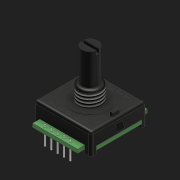
# Autodesk Inventor part: Bourns ACE 128
Saved by Autodesk Inventor 2017 SP1 (Build 210196100, 196)
## iProperties
Created: 2018-01-09
Part Number: Bourns ACE 128
Material: ABS Plastic
Document SubType Name: Modeling
Designer: Zach
Density: 1.06 g/cm^3
Appearance: Glossy - Black
Author: Zach
Autodesk Inventor part; units mm, degrees
ref_plane "YZ Plane" through (0, 0, 0) normal (1, 0, 0) x (0, 1, 0)
ref_plane "XZ Plane" through (0, 0, 0) normal (0, 1, 0) x (-1, 0, 0)
sketch "Sketch1" plane through (0, 0, 0) normal (0, 0, 1) x (1, 0, 0)
  line L0 (0, 0) -> (18.04, 0)
  line L1 (18.04, 0) -> (18.04, 27.94) construction
  line L2 (18.04, 27.94) -> (0, 27.94)
  line L3 (0, 27.94) -> (0, 0) construction
  circle A0 centre (9.02, 26.94) radius 0.32
  circle A1 centre (6.48, 26.94) radius 0.32
  circle A2 centre (3.94, 26.94) radius 0.32
  circle A3 centre (11.56, 26.94) radius 0.32
  circle A4 centre (14.1, 26.94) radius 0.32
  circle A5 centre (9.02, 1) radius 0.32
  circle A6 centre (6.48, 1) radius 0.32
  circle A7 centre (3.94, 1) radius 0.32
  circle A8 centre (11.56, 1) radius 0.32
  circle A9 centre (14.1, 1) radius 0.32
  line L4 (-2.665, 23.07) -> (20.705, 23.07) construction
  line L5 (20.705, 23.07) -> (20.705, 4.87) construction
  line L6 (20.705, 4.87) -> (-2.665, 4.87) construction
  line L7 (-2.665, 4.87) -> (-2.665, 23.07) construction
  line L8 (0, 27.94) -> (0, 23.07)
  line L9 (0, 23.07) -> (-2.665, 23.07)
  line L10 (-2.665, 23.07) -> (-2.665, 4.87)
  line L11 (-2.665, 4.87) -> (0, 4.87)
  line L12 (0, 0) -> (0, 4.87)
  line L13 (18.04, 0) -> (18.04, 4.87)
  line L14 (18.04, 4.87) -> (20.705, 4.87)
  line L15 (20.705, 4.87) -> (20.705, 23.07)
  line L16 (20.705, 23.07) -> (18.04, 23.07)
  line L17 (18.04, 23.07) -> (18.04, 27.94)
  point P0 (9.02, 27.94)
  point P1 (9.02, 23.07)
  point P2 (18.04, 13.97)
  point P3 (20.705, 13.97)
  dimension "d0" = 18.04
  dimension "d1" = 27.94
  dimension "d2" = 0.64
  dimension "d3" = 0.64
  dimension "d4" = 2.54
  dimension "d5" = 0.64
  dimension "d6" = 0.64
  dimension "d7" = 0.64
  dimension "d8" = 2.54
  dimension "d9" = 2.54
  dimension "d10" = 2.54
  dimension "d11" = 1
  dimension "d12" = 0.64
  dimension "d13" = 0.64
  dimension "d14" = 2.54
  dimension "d15" = 0.64
  dimension "d16" = 0.64
  dimension "d17" = 0.64
  dimension "d18" = 2.54
  dimension "d19" = 2.54
  dimension "d20" = 2.54
  dimension "d21" = 1
  dimension "d24" = 23.37
  dimension "d25" = 18.2
  constraints: 36 end point, 10 centre point, 9 horizontal alignment, 8 point on line, 4 collinear, 4 midpoint, 4 parallel, 4 perpendicular, 3 vertical alignment, 2 horizontal
  measures "d0" distance of L2.end L1.end
  measures "d1" distance of L1.end L0.end
  measures "d2" diameter of A0
  measures "d3" diameter of A1
  measures "d4" distance of A0.centre A1.centre
  measures "d5" diameter of A2
  measures "d6" diameter of A3
  measures "d7" diameter of A4
  measures "d8" distance of A3.centre A0.centre
  measures "d9" distance of A4.centre A3.centre
  measures "d10" distance of A2.centre A1.centre
  measures "d11" distance from line of L2 A2.centre
  measures "d12" diameter of A5
  measures "d13" diameter of A6
  measures "d14" distance of A5.centre A6.centre
  measures "d15" diameter of A7
  measures "d16" diameter of A8
  measures "d17" diameter of A9
  measures "d18" distance of A8.centre A5.centre
  measures "d19" distance of A9.centre A8.centre
  measures "d20" distance of A7.centre A6.centre
  measures "d21" distance from line of L0 A5.centre
  measures "d24" distance of L5.end L6.end
  measures "d25" distance of L4.end L5.end
extrude "Extrusion1" add sketch "Sketch1" along normal blind 1.5
sketch "Sketch2" plane through (0, 0, 1.5) normal (0, 0, 1) x (1, 0, 0)
  line L0 (-2.565, 25.07) -> (20.605, 25.07)
  line L1 (20.605, 25.07) -> (20.605, 2.87)
  line L2 (20.605, 2.87) -> (-2.565, 2.87)
  line L3 (-2.565, 2.87) -> (-2.565, 25.07)
  line L4 (-2.665, 23.07) -> (-2.665, 4.87) projected
  line L5 (20.705, 4.87) -> (20.705, 23.07) projected
  line L6 (18.04, 27.94) -> (0, 27.94) projected
  point P0 (0, 0)
  point P1 (9.02, 25.07)
  point P2 (9.02, 27.94)
  dimension "d27" = 22.2
  dimension "d30" = 0.1
  constraints: 8 end point, 2 midpoint, 2 parallel, 1 horizontal, 1 perpendicular, 1 vertical alignment
  measures "d27" distance of L0.end L1.end
  measures "d30" distance between parallel lines of L5 L1
extrude "Extrusion2" add sketch "Sketch2" along normal blind 5.51
sketch "Sketch3" plane through (0, 0, 1.5) normal (0, 0, -1) x (-1, 0, 0)
  line L0 (0, 23.07) -> (2.565, 23.07) projected
  line L1 (2.565, 23.07) -> (2.565, 25.07) projected
  line L2 (2.565, 25.07) -> (0, 25.07) projected
  line L3 (0, 25.07) -> (0, 23.07) projected
  line L4 (0, 4.87) -> (0, 2.87) projected
  line L5 (0, 2.87) -> (2.565, 2.87) projected
  line L6 (2.565, 2.87) -> (2.565, 4.87) projected
  line L7 (2.565, 4.87) -> (0, 4.87) projected
  line L8 (-20.605, 23.07) -> (-18.04, 23.07) projected
  line L9 (-18.04, 23.07) -> (-18.04, 25.07) projected
  line L10 (-18.04, 25.07) -> (-20.605, 25.07) projected
  line L11 (-20.605, 25.07) -> (-20.605, 23.07) projected
  line L12 (-18.04, 2.87) -> (-18.04, 4.87) projected
  line L13 (-18.04, 4.87) -> (-20.605, 4.87) projected
  line L14 (-20.605, 4.87) -> (-20.605, 2.87) projected
  line L15 (-20.605, 2.87) -> (-18.04, 2.87) projected
  point P0 (0, 0)
extrude "Extrusion3" add sketch "Sketch3" along normal blind 3
sketch "Sketch4" plane through (0, 0, 7.01) normal (0, 0, 1) x (1, 0, 0)
  circle A0 centre (9.02, 13.97) radius 4.5
  line L0 (20.605, 25.07) -> (-2.565, 25.07) construction
  line L1 (-2.565, 25.07) -> (-2.565, 2.87) construction
  line L2 (-2.565, 2.87) -> (20.605, 2.87) construction
  line L3 (20.605, 2.87) -> (20.605, 25.07) construction
  point P0 (0, 0)
  point P1 (9.02, 25.07)
  point P2 (20.605, 13.97)
  dimension "d33" = 9
  constraints: 2 midpoint, 1 centre point, 1 horizontal alignment, 1 vertical alignment
  measures "d33" diameter of A0
extrude "Extrusion4" add sketch "Sketch4" along normal blind 6.35
sketch "Sketch5" plane through (9.02, 13.97, 13.36) normal (0, 0, 1) x (1, 0, 0)
  circle A0 centre (0, 0) radius 3.16
  circle A1 centre (0, 0) radius 4.5 construction
  point P0 (-9.02, -13.97)
  dimension "d36" = 6.32
  constraints: 1 centre point, 1 coincident
  measures "d36" diameter of A0
extrude "Extrusion5" add sketch "Sketch5" along normal blind 12.7
sketch "Sketch6" plane through (9.02, 13.97, 26.06) normal (0, 0, 1) x (1, 0, 0)
  line L0 (-3.16, 0.595) -> (3.16, 0.595)
  line L1 (3.16, 0.595) -> (3.16, -0.595)
  line L2 (3.16, -0.595) -> (-3.16, -0.595)
  line L3 (-3.16, -0.595) -> (-3.16, 0.595)
  circle A0 centre (0, 0) radius 3.16 construction
  point P0 (-9.02, -13.97)
  point P1 (3.16, 0)
  point P2 (0, 0.595)
  dimension "d39" = 1.19
  constraints: 8 end point, 2 horizontal alignment, 2 midpoint, 2 parallel, 1 horizontal, 1 perpendicular, 1 vertical alignment, 1 other
  measures "d39" distance of L0.end L1.end
extrude "Extrusion6" cut sketch "Sketch6" against normal blind 1.6
thread "Thread1" size "M9x1.25" class "6g" standard "ANSI Metric M Profile" full length
fillet "Fillet1" radius 1 1 edges at (4.52, 13.97, 13.36)
fillet "Fillet2" radius 1 4 edges at (20.605, 2.87, 2.755) (-2.565, 2.87, 2.755) (-2.565, 25.07, 2.755) (20.605, 25.07, 2.755)
fillet "Fillet3" radius 1 8 edges at (-2.2721, 24.7771, 7.01) (-2.565, 13.97, 7.01) (-2.2721, 3.1629, 7.01) (9.02, 2.87, 7.01) (20.3121, 3.1629, 7.01) (20.605, 13.97, 7.01) (20.3121, 24.7771, 7.01) (9.02, 25.07, 7.01)
ref_plane "Work Plane1" through (0, 13.97, 1.5) normal (0, 1, 0) x (1, 0, 0)
sketch "Sketch8" plane through (0, 13.97, 1.5) normal (0, 1, 0) x (1, 0, 0)
  line L0 (19.605, -1.51) -> (21.605, -1.51)
  line L1 (19.605, 3) -> (19.605, -4.51) construction
  line L2 (19.605, -1.51) -> (19.605, -5.51)
  line L3 (0, 1.5) -> (18.04, 1.5) construction
  line L4 (9.02, 1.5) -> (9.02, -5.51) construction
  line L5 (19.605, -5.51) -> (-1.565, -5.51) construction
  line L6 (21.605, -1.51) -> (19.605, -5.51)
  line L7 (-1.565, -1.51) -> (-3.565, -1.51)
  line L8 (-1.565, -1.51) -> (-1.565, -5.51)
  line L9 (-3.565, -1.51) -> (-1.565, -5.51)
  dimension "d47" = 2
  dimension "d48" = 4
  constraints: 14 end point, 3 symmetric about line, 2 vertical, 1 horizontal, 1 midpoint, 1 point on line
  measures "d47" distance of L0.start L0.end
  measures "d48" distance of L2.end L0.start
extrude "Extrusion7" add sketch "Sketch8" along normal mid plane 2.79
sketch "Sketch9" plane through (0, 13.97, 1.5) normal (0, 1, 0) x (1, 0, 0)
  line L0 (-1.565, -5.51) -> (19.605, -5.51) projected
  line L1 (19.605, -5.51) -> (18.415, -5.51)
  line L2 (18.415, -5.51) -> (18.415, -7.03)
  line L3 (18.415, -7.03) -> (19.605, -7.03)
  line L4 (19.605, -7.03) -> (19.605, -5.51)
  point P0 (0, 1.5)
  dimension "d51" = 1.52
  dimension "d52" = 1.19
  constraints: 8 end point, 2 parallel, 1 horizontal, 1 perpendicular
  measures "d51" distance of L2.end L1.end
  measures "d52" distance of L2.end L3.end
extrude "Extrusion8" add sketch "Sketch9" along normal mid plane 2.79
sketch "Sketch10" plane through (0, 0, 7.01) normal (0, 0, 1) x (1, 0, 0)
  circle A0 centre (9.02, 13.97) radius 4.5 projected
  circle A1 centre (9.02, 13.97) radius 7.35
  point P0 (0, 0)
  dimension "d55" = 14.7
  constraints: 1 centre point, 1 coincident
  measures "d55" diameter of A1
extrude "Extrusion9" add sketch "Sketch10" along normal blind 0.25 contours A0 | A1
sketch "Sketch11" plane through (0, 0, 1.5) normal (0, 0, 1) x (1, 0, 0)
  circle A0 centre (9.02, 1) radius 0.32 projected
  circle A1 centre (6.48, 1) radius 0.32 projected
  circle A2 centre (3.94, 1) radius 0.32 projected
  circle A3 centre (11.56, 1) radius 0.32 projected
  circle A4 centre (14.1, 1) radius 0.32 projected
  line L0 (18.04, 2.87) -> (0, 2.87) projected
  line L1 (0, 2.87) -> (0, 0) construction
  line L2 (0, 0) -> (18.04, 0) construction
  line L3 (18.04, 0) -> (18.04, 2.87) construction
  circle A5 centre (9.02, 26.94) radius 0.32 projected
  circle A6 centre (6.48, 26.94) radius 0.32 projected
  circle A7 centre (3.94, 26.94) radius 0.32 projected
  circle A8 centre (11.56, 26.94) radius 0.32 projected
  circle A9 centre (14.1, 26.94) radius 0.32 projected
  line L4 (0, 25.07) -> (18.04, 25.07) construction
  line L5 (18.04, 25.07) -> (18.04, 27.94) construction
  line L6 (18.04, 27.94) -> (0, 27.94) construction
  line L7 (0, 27.94) -> (0, 25.07) construction
extrude "Extrusion10" add sketch "Sketch11" along normal blind 1 and the other way blind 6.5
sketch "Sketch12" plane through (0, 0, 7.01) normal (0, 0, 1) x (1, 0, 0)
  line L0 (16.6233, 23.2524) -> (16.6233, 21.4375) construction
  line L1 (16.6233, 21.4375) -> (0.9162, 21.4375) construction
  line L2 (0.9162, 21.4375) -> (0.9162, 23.2524) construction
  line L3 (0.9162, 23.2524) -> (16.6233, 23.2524) construction
  line L4 (16.6326, 7.0655) -> (16.6326, 4.3638) construction
  line L5 (16.6326, 4.3638) -> (0.3771, 4.3638) construction
  line L6 (0.3771, 4.3638) -> (0.3771, 7.0655) construction
  line L7 (0.3771, 7.0655) -> (16.6326, 7.0655) construction
  line L8 (14.592, 6.0867) -> (14.592, 7.0623)
  line L9 (14.592, 7.0623) -> (14.7963, 7.0623)
  line L10 (14.7963, 7.0623) -> (14.7963, 6.6993)
  line L11 (14.7963, 6.6993) -> (16.1366, 6.6993)
  line L12 (16.1366, 6.6993) -> (16.1366, 7.0623)
  line L13 (16.1366, 7.0623) -> (16.3198, 7.0623)
  spline S0 degree 2 poles (16.3198, 7.0623) (16.3198, 6.8565) (16.4365, 6.662) (16.5985, 6.6491) knots 0 0 0 1 2 2 2
  line L14 (16.5985, 6.6491) -> (16.5985, 6.4416)
  line L15 (16.5985, 6.4416) -> (14.7963, 6.4416)
  line L16 (14.7963, 6.4416) -> (14.7963, 6.0867)
  line L17 (14.7963, 6.0867) -> (14.592, 6.0867)
  spline S1 degree 2 poles (15.592, 4.474) (15.054, 4.474) (14.5499, 4.7868) (14.5499, 5.1126) knots 0 0 0 1 2 2 2
  spline S2 degree 2 poles (14.5499, 5.1126) (14.5499, 5.4432) (15.0637, 5.7528) (15.5904, 5.7528) knots 0 0 0 1 2 2 2
  spline S3 degree 2 poles (15.5904, 5.7528) (16.1318, 5.7528) (16.6326, 5.44) (16.6326, 5.1126) knots 0 0 0 1 2 2 2
  spline S4 degree 2 poles (16.6326, 5.1126) (16.6326, 4.7836) (16.1139, 4.474) (15.592, 4.474) knots 0 0 0 1 2 2 2
  spline S5 degree 2 poles (14.9826, 4.8176) (15.0815, 4.7787) (15.3862, 4.7463) (15.592, 4.7463) knots 0 0 0 1 2 2 2
  spline S6 degree 2 poles (15.592, 4.7463) (15.7979, 4.7463) (16.101, 4.7787) (16.2031, 4.8192) knots 0 0 0 1 2 2 2
  spline S7 degree 2 poles (16.2031, 4.8192) (16.3052, 4.8598) (16.4105, 5.0008) (16.4105, 5.1126) knots 0 0 0 1 2 2 2
  spline S8 degree 2 poles (16.4105, 5.1126) (16.4105, 5.2244) (16.3052, 5.3687) (16.1998, 5.4108) knots 0 0 0 1 2 2 2
  spline S9 degree 2 poles (16.1998, 5.4108) (16.0977, 5.4513) (15.7865, 5.4805) (15.5904, 5.4805) knots 0 0 0 1 2 2 2
  spline S10 degree 2 poles (15.5904, 5.4805) (15.3797, 5.4805) (15.0977, 5.4546) (14.9875, 5.4124) knots 0 0 0 1 2 2 2
  spline S11 degree 2 poles (14.9875, 5.4124) (14.8838, 5.3735) (14.7719, 5.2293) (14.7719, 5.1126) knots 0 0 0 1 2 2 2
  spline S12 degree 2 poles (14.7719, 5.1126) (14.7719, 5.0024) (14.8773, 4.8581) (14.9826, 4.8176) knots 0 0 0 1 2 2 2
  spline S13 degree 2 poles (12.6492, 5.7739) (12.8031, 5.7739) (13.0592, 5.6734) (13.1516, 5.5858) knots 0 0 0 1 2 2 2
  spline S14 degree 2 poles (13.1516, 5.5858) (13.2407, 5.5032) (13.3396, 5.2617) (13.3396, 5.1385) knots 0 0 0 1 2 2 2
  spline S15 degree 2 poles (13.3396, 5.1385) (13.3396, 5.0008) (13.2472, 4.7771) (13.1597, 4.6944) knots 0 0 0 1 2 2 2
  spline S16 degree 2 poles (13.1597, 4.6944) (13.0495, 4.5907) (12.6929, 4.4773) (12.419, 4.4773) knots 0 0 0 1 2 2 2
  spline S17 degree 2 poles (12.419, 4.4773) (12.1711, 4.4773) (11.727, 4.5891) (11.5795, 4.6977) knots 0 0 0 1 2 2 2
  spline S18 degree 2 poles (11.5795, 4.6977) (11.4239, 4.8127) (11.2602, 5.1369) (11.2602, 5.3735) knots 0 0 0 1 2 2 2
  spline S19 degree 2 poles (11.2602, 5.3735) (11.2602, 5.427) (11.2715, 5.5486) (11.2877, 5.6004) knots 0 0 0 1 2 2 2
  line L18 (11.2877, 5.6004) -> (11.5454, 5.6004)
  line L19 (11.5454, 5.6004) -> (11.5454, 5.5875)
  spline S20 degree 2 poles (11.5454, 5.5875) (11.526, 5.5534) (11.492, 5.4108) (11.492, 5.3379) knots 0 0 0 1 2 2 2
  spline S21 degree 2 poles (11.492, 5.3379) (11.492, 5.0753) (11.8388, 4.7755) (12.1597, 4.7544) knots 0 0 0 1 2 2 2
  spline S22 degree 2 poles (12.1597, 4.7544) (12.0868, 4.8614) (12.0203, 5.0559) (12.0203, 5.1709) knots 0 0 0 1 2 2 2
  spline S23 degree 2 poles (12.0203, 5.1709) (12.0203, 5.2811) (12.0689, 5.4643) (12.1386, 5.5567) knots 0 0 0 1 2 2 2
  spline S24 degree 2 poles (12.1386, 5.5567) (12.2213, 5.6636) (12.4725, 5.7739) (12.6492, 5.7739) knots 0 0 0 1 2 2 2
  spline S25 degree 2 poles (12.479, 4.7479) (12.6816, 4.7479) (12.9377, 4.8225) (13.0074, 4.8889) knots 0 0 0 1 2 2 2
  spline S26 degree 2 poles (13.0074, 4.8889) (13.0722, 4.9473) (13.1208, 5.0688) (13.1208, 5.1401) knots 0 0 0 1 2 2 2
  spline S27 degree 2 poles (13.1208, 5.1401) (13.1208, 5.3055) (12.8842, 5.5016) (12.6605, 5.5016) knots 0 0 0 1 2 2 2
  spline S28 degree 2 poles (12.6605, 5.5016) (12.5341, 5.5016) (12.3704, 5.4367) (12.3121, 5.3654) knots 0 0 0 1 2 2 2
  spline S29 degree 2 poles (12.3121, 5.3654) (12.2699, 5.3136) (12.2424, 5.1855) (12.2424, 5.111) knots 0 0 0 1 2 2 2
  spline S30 degree 2 poles (12.2424, 5.111) (12.2424, 5.0251) (12.3023, 4.8273) (12.3526, 4.7528) knots 0 0 0 1 2 2 2
  spline S31 degree 2 poles (12.3526, 4.7528) (12.372, 4.7512) (12.4385, 4.7479) (12.479, 4.7479) knots 0 0 0 1 2 2 2
  spline S32 degree 2 poles (7.9608, 5.1142) (7.9608, 5.2633) (8.0499, 5.508) (8.1326, 5.5939) knots 0 0 0 1 2 2 2
  spline S33 degree 2 poles (8.1326, 5.5939) (8.2136, 5.6782) (8.434, 5.7657) (8.5588, 5.7657) knots 0 0 0 1 2 2 2
  spline S34 degree 2 poles (8.5588, 5.7657) (8.7209, 5.7657) (8.9932, 5.5923) (9.0742, 5.427) knots 0 0 0 1 2 2 2
  line L20 (9.0742, 5.427) -> (9.0823, 5.427)
  spline S35 degree 2 poles (9.0823, 5.427) (9.1682, 5.5745) (9.3724, 5.7171) (9.5248, 5.7171) knots 0 0 0 1 2 2 2
  spline S36 degree 2 poles (9.5248, 5.7171) (9.7501, 5.7171) (10.0515, 5.3768) (10.0515, 5.1142) knots 0 0 0 1 2 2 2
  spline S37 degree 2 poles (10.0515, 5.1142) (10.0515, 4.8419) (9.7663, 4.5129) (9.5426, 4.5129) knots 0 0 0 1 2 2 2
  spline S38 degree 2 poles (9.5426, 4.5129) (9.4081, 4.5129) (9.1455, 4.6701) (9.071, 4.8176) knots 0 0 0 1 2 2 2
  line L21 (9.071, 4.8176) -> (9.0629, 4.8176)
  spline S39 degree 2 poles (9.0629, 4.8176) (8.9818, 4.6426) (8.7484, 4.4627) (8.5637, 4.4627) knots 0 0 0 1 2 2 2
  spline S40 degree 2 poles (8.5637, 4.4627) (8.3076, 4.4627) (7.9608, 4.8354) (7.9608, 5.1142) knots 0 0 0 1 2 2 2
  spline S41 degree 2 poles (8.5378, 4.7382) (8.6609, 4.7382) (8.8068, 4.8354) (8.8814, 4.9732) knots 0 0 0 1 2 2 2
  spline S42 degree 2 poles (8.8814, 4.9732) (8.9073, 5.0186) (8.9673, 5.1709) (9.0061, 5.2666) knots 0 0 0 1 2 2 2
  spline S43 degree 2 poles (9.0061, 5.2666) (8.9332, 5.3768) (8.716, 5.4951) (8.5783, 5.4951) knots 0 0 0 1 2 2 2
  spline S44 degree 2 poles (8.5783, 5.4951) (8.3967, 5.4951) (8.1601, 5.2763) (8.1601, 5.111) knots 0 0 0 1 2 2 2
  spline S45 degree 2 poles (8.1601, 5.111) (8.1601, 4.9424) (8.3627, 4.7382) (8.5378, 4.7382) knots 0 0 0 1 2 2 2
  spline S46 degree 2 poles (9.5394, 4.7755) (9.6739, 4.7755) (9.8538, 4.9554) (9.8538, 5.1158) knots 0 0 0 1 2 2 2
  spline S47 degree 2 poles (9.8538, 5.1158) (9.8538, 5.2617) (9.6933, 5.4481) (9.5556, 5.4481) knots 0 0 0 1 2 2 2
  spline S48 degree 2 poles (9.5556, 5.4481) (9.4567, 5.4481) (9.319, 5.3525) (9.2638, 5.2568) knots 0 0 0 1 2 2 2
  spline S49 degree 2 poles (9.2638, 5.2568) (9.2412, 5.2163) (9.1617, 5.0445) (9.139, 4.9748) knots 0 0 0 1 2 2 2
  spline S50 degree 2 poles (9.139, 4.9748) (9.2282, 4.8581) (9.4178, 4.7755) (9.5394, 4.7755) knots 0 0 0 1 2 2 2
  line L22 (6.4134, 4.4627) -> (4.7132, 5.3281)
  line L23 (4.7132, 5.3281) -> (4.7132, 5.6134)
  line L24 (4.7132, 5.6134) -> (6.4782, 4.6993)
  line L25 (6.4782, 4.6993) -> (6.4782, 5.7317)
  line L26 (6.4782, 5.7317) -> (6.7132, 5.7317)
  line L27 (6.7132, 5.7317) -> (6.7132, 4.4627)
  line L28 (6.7132, 4.4627) -> (6.4134, 4.4627)
  spline S51 degree 2 poles (2.0686, 4.4546) (1.9146, 4.4546) (1.6536, 4.5567) (1.5661, 4.6426) knots 0 0 0 1 2 2 2
  spline S52 degree 2 poles (1.5661, 4.6426) (1.4737, 4.7317) (1.3781, 4.9554) (1.3781, 5.0899) knots 0 0 0 1 2 2 2
  spline S53 degree 2 poles (1.3781, 5.0899) (1.3781, 5.2244) (1.4689, 5.4465) (1.5596, 5.5307) knots 0 0 0 1 2 2 2
  spline S54 degree 2 poles (1.5596, 5.5307) (1.6682, 5.6345) (2.0329, 5.7512) (2.2987, 5.7512) knots 0 0 0 1 2 2 2
  spline S55 degree 2 poles (2.2987, 5.7512) (2.5596, 5.7512) (2.9794, 5.6442) (3.135, 5.5324) knots 0 0 0 1 2 2 2
  spline S56 degree 2 poles (3.135, 5.5324) (3.2874, 5.4238) (3.4575, 5.0802) (3.4575, 4.8549) knots 0 0 0 1 2 2 2
  spline S57 degree 2 poles (3.4575, 4.8549) (3.4575, 4.7884) (3.4446, 4.6717) (3.43, 4.628) knots 0 0 0 1 2 2 2
  line L29 (3.43, 4.628) -> (3.1723, 4.628)
  line L30 (3.1723, 4.628) -> (3.1723, 4.6393)
  spline S58 degree 2 poles (3.1723, 4.6393) (3.1917, 4.6766) (3.2258, 4.8127) (3.2258, 4.8905) knots 0 0 0 1 2 2 2
  spline S59 degree 2 poles (3.2258, 4.8905) (3.2258, 5.1401) (2.8886, 5.4465) (2.558, 5.4756) knots 0 0 0 1 2 2 2
  spline S60 degree 2 poles (2.558, 5.4756) (2.6245, 5.38) (2.6974, 5.179) (2.6974, 5.0591) knots 0 0 0 1 2 2 2
  spline S61 degree 2 poles (2.6974, 5.0591) (2.6974, 4.9424) (2.6504, 4.7674) (2.5791, 4.6717) knots 0 0 0 1 2 2 2
  spline S62 degree 2 poles (2.5791, 4.6717) (2.4964, 4.5615) (2.2404, 4.4546) (2.0686, 4.4546) knots 0 0 0 1 2 2 2
  spline S63 degree 2 poles (2.0572, 4.7269) (2.1804, 4.7269) (2.3473, 4.7917) (2.4057, 4.863) knots 0 0 0 1 2 2 2
  spline S64 degree 2 poles (2.4057, 4.863) (2.4478, 4.9165) (2.4754, 5.0494) (2.4754, 5.1191) knots 0 0 0 1 2 2 2
  spline S65 degree 2 poles (2.4754, 5.1191) (2.4754, 5.2131) (2.4186, 5.3897) (2.3651, 5.4756) knots 0 0 0 1 2 2 2
  spline S66 degree 2 poles (2.3651, 5.4756) (2.336, 5.4773) (2.2809, 5.4805) (2.2387, 5.4805) knots 0 0 0 1 2 2 2
  spline S67 degree 2 poles (2.2387, 5.4805) (2.0313, 5.4805) (1.7768, 5.3995) (1.7104, 5.3379) knots 0 0 0 1 2 2 2
  spline S68 degree 2 poles (1.7104, 5.3379) (1.6472, 5.2811) (1.5969, 5.158) (1.5969, 5.0883) knots 0 0 0 1 2 2 2
  spline S69 degree 2 poles (1.5969, 5.0883) (1.5969, 4.9262) (1.8271, 4.7269) (2.0572, 4.7269) knots 0 0 0 1 2 2 2
  line L31 (14.6168, 21.9736) -> (14.6168, 22.9493)
  line L32 (14.6168, 22.9493) -> (14.821, 22.9493)
  line L33 (14.821, 22.9493) -> (14.821, 22.5863)
  line L34 (14.821, 22.5863) -> (16.1614, 22.5863)
  line L35 (16.1614, 22.5863) -> (16.1614, 22.9493)
  line L36 (16.1614, 22.9493) -> (16.3445, 22.9493)
  spline S70 degree 2 poles (16.3445, 22.9493) (16.3445, 22.7435) (16.4612, 22.549) (16.6233, 22.536) knots 0 0 0 1 2 2 2
  line L37 (16.6233, 22.536) -> (16.6233, 22.3286)
  line L38 (16.6233, 22.3286) -> (14.821, 22.3286)
  line L39 (14.821, 22.3286) -> (14.821, 21.9736)
  line L40 (14.821, 21.9736) -> (14.6168, 21.9736)
  line L41 (11.3238, 21.8731) -> (11.3238, 23.1065)
  line L42 (11.3238, 23.1065) -> (11.6075, 23.1065)
  spline S71 degree 2 poles (11.6075, 23.1065) (11.7323, 22.9736) (11.964, 22.737) (12.0888, 22.6236) knots 0 0 0 1 2 2 2
  spline S72 degree 2 poles (12.0888, 22.6236) (12.34, 22.395) (12.6415, 22.2281) (12.802, 22.2281) knots 0 0 0 1 2 2 2
  spline S73 degree 2 poles (12.802, 22.2281) (12.8862, 22.2281) (13.0127, 22.28) (13.0532, 22.327) knots 0 0 0 1 2 2 2
  spline S74 degree 2 poles (13.0532, 22.327) (13.0937, 22.374) (13.1342, 22.4971) (13.1342, 22.5717) knots 0 0 0 1 2 2 2
  spline S75 degree 2 poles (13.1342, 22.5717) (13.1342, 22.643) (13.0986, 22.7889) (13.071, 22.8553) knots 0 0 0 1 2 2 2
  spline S76 degree 2 poles (13.071, 22.8553) (13.0483, 22.912) (12.9835, 23.0174) (12.9608, 23.0498) knots 0 0 0 1 2 2 2
  line L43 (12.9608, 23.0498) -> (12.9608, 23.0644)
  line L44 (12.9608, 23.0644) -> (13.246, 23.0644)
  spline S77 degree 2 poles (13.246, 23.0644) (13.2866, 22.9817) (13.366, 22.6851) (13.366, 22.5522) knots 0 0 0 1 2 2 2
  spline S78 degree 2 poles (13.366, 22.5522) (13.366, 22.2718) (13.0694, 21.9558) (12.8165, 21.9558) knots 0 0 0 1 2 2 2
  spline S79 degree 2 poles (12.8165, 21.9558) (12.6982, 21.9558) (12.5005, 22.0109) (12.4162, 22.0595) knots 0 0 0 1 2 2 2
  spline S80 degree 2 poles (12.4162, 22.0595) (12.3287, 22.1082) (12.1569, 22.2492) (12.0742, 22.327) knots 0 0 0 1 2 2 2
  spline S81 degree 2 poles (12.0742, 22.327) (11.9365, 22.4534) (11.6415, 22.7629) (11.5556, 22.8553) knots 0 0 0 1 2 2 2
  line L45 (11.5556, 22.8553) -> (11.5556, 21.8731)
  line L46 (11.5556, 21.8731) -> (11.3238, 21.8731)
  spline S82 degree 2 poles (9.8413, 22.5668) (9.8413, 22.6398) (9.8056, 22.784) (9.7781, 22.8537) knots 0 0 0 1 2 2 2
  spline S83 degree 2 poles (9.7781, 22.8537) (9.7505, 22.9185) (9.6922, 23.0142) (9.6662, 23.0514) knots 0 0 0 1 2 2 2
  line L47 (9.6662, 23.0514) -> (9.6662, 23.0676)
  line L48 (9.6662, 23.0676) -> (9.9498, 23.0676)
  spline S84 degree 2 poles (9.9498, 23.0676) (9.9969, 22.9801) (10.073, 22.6803) (10.073, 22.5458) knots 0 0 0 1 2 2 2
  spline S85 degree 2 poles (10.073, 22.5458) (10.073, 22.4096) (10.0179, 22.207) (9.9596, 22.1244) knots 0 0 0 1 2 2 2
  spline S86 degree 2 poles (9.9596, 22.1244) (9.8964, 22.0368) (9.7132, 21.9461) (9.59, 21.9461) knots 0 0 0 1 2 2 2
  spline S87 degree 2 poles (9.59, 21.9461) (9.4247, 21.9461) (9.1751, 22.1633) (9.1427, 22.3156) knots 0 0 0 1 2 2 2
  line L49 (9.1427, 22.3156) -> (9.1233, 22.3156)
  spline S88 degree 2 poles (9.1233, 22.3156) (9.1103, 22.2524) (9.052, 22.1082) (8.9936, 22.0466) knots 0 0 0 1 2 2 2
  spline S89 degree 2 poles (8.9936, 22.0466) (8.9369, 21.985) (8.7554, 21.9072) (8.6241, 21.9072) knots 0 0 0 1 2 2 2
  spline S90 degree 2 poles (8.6241, 21.9072) (8.4896, 21.9072) (8.261, 21.9996) (8.1735, 22.0838) knots 0 0 0 1 2 2 2
  spline S91 degree 2 poles (8.1735, 22.0838) (8.0828, 22.1714) (7.9887, 22.4193) (7.9887, 22.5765) knots 0 0 0 1 2 2 2
  spline S92 degree 2 poles (7.9887, 22.5765) (7.9887, 22.7273) (8.0617, 23.0223) (8.1119, 23.1227) knots 0 0 0 1 2 2 2
  line L50 (8.1119, 23.1227) -> (8.3956, 23.1227)
  line L51 (8.3956, 23.1227) -> (8.3956, 23.1033)
  spline S93 degree 2 poles (8.3956, 23.1033) (8.334, 23.019) (8.2205, 22.7338) (8.2205, 22.5928) knots 0 0 0 1 2 2 2
  spline S94 degree 2 poles (8.2205, 22.5928) (8.2205, 22.5101) (8.2724, 22.3448) (8.3323, 22.2897) knots 0 0 0 1 2 2 2
  spline S95 degree 2 poles (8.3323, 22.2897) (8.3923, 22.2362) (8.5349, 22.1795) (8.6435, 22.1795) knots 0 0 0 1 2 2 2
  spline S96 degree 2 poles (8.6435, 22.1795) (8.7521, 22.1795) (8.8931, 22.2427) (8.9336, 22.2994) knots 0 0 0 1 2 2 2
  spline S97 degree 2 poles (8.9336, 22.2994) (8.9742, 22.3561) (9.005, 22.5101) (9.005, 22.6009) knots 0 0 0 1 2 2 2
  line L52 (9.005, 22.6009) -> (9.005, 22.7143)
  line L53 (9.005, 22.7143) -> (9.227, 22.7143)
  line L54 (9.227, 22.7143) -> (9.227, 22.6252)
  spline S98 degree 2 poles (9.227, 22.6252) (9.227, 22.4453) (9.3988, 22.2184) (9.5625, 22.2184) knots 0 0 0 1 2 2 2
  spline S99 degree 2 poles (9.5625, 22.2184) (9.6387, 22.2184) (9.7473, 22.2767) (9.7797, 22.3237) knots 0 0 0 1 2 2 2
  spline S100 degree 2 poles (9.7797, 22.3237) (9.8137, 22.374) (9.8413, 22.4971) (9.8413, 22.5668) knots 0 0 0 1 2 2 2
  line L55 (5.4251, 21.8197) -> (5.4251, 22.0579)
  line L56 (5.4251, 22.0579) -> (4.7379, 22.0579)
  line L57 (4.7379, 22.0579) -> (4.7379, 22.3156)
  line L58 (4.7379, 22.3156) -> (5.4251, 22.3156)
  line L59 (5.4251, 22.3156) -> (5.4251, 23.1989)
  line L60 (5.4251, 23.1989) -> (5.7071, 23.1989)
  line L61 (5.7071, 23.1989) -> (6.7379, 22.3043)
  line L62 (6.7379, 22.3043) -> (6.7379, 22.0579)
  line L63 (6.7379, 22.0579) -> (5.6407, 22.0579)
  line L64 (5.6407, 22.0579) -> (5.6407, 21.8197)
  line L65 (5.6407, 21.8197) -> (5.4251, 21.8197)
  line L66 (5.6407, 22.3156) -> (6.4219, 22.3156)
  line L67 (6.4219, 22.3156) -> (5.6407, 22.9882)
  line L68 (5.6407, 22.9882) -> (5.6407, 22.3156)
  spline S101 degree 2 poles (2.0803, 21.8942) (1.9361, 21.8942) (1.6897, 21.9866) (1.599, 22.0709) knots 0 0 0 1 2 2 2
  spline S102 degree 2 poles (1.599, 22.0709) (1.5082, 22.1552) (1.4029, 22.4064) (1.4029, 22.562) knots 0 0 0 1 2 2 2
  spline S103 degree 2 poles (1.4029, 22.562) (1.4029, 22.7046) (1.4661, 22.9834) (1.5163, 23.0855) knots 0 0 0 1 2 2 2
  line L69 (1.5163, 23.0855) -> (1.7999, 23.0855)
  line L70 (1.7999, 23.0855) -> (1.7999, 23.066)
  spline S104 degree 2 poles (1.7999, 23.066) (1.7772, 23.0352) (1.7189, 22.9201) (1.693, 22.8505) knots 0 0 0 1 2 2 2
  spline S105 degree 2 poles (1.693, 22.8505) (1.6654, 22.771) (1.6346, 22.6398) (1.6346, 22.5571) knots 0 0 0 1 2 2 2
  spline S106 degree 2 poles (1.6346, 22.5571) (1.6346, 22.4761) (1.693, 22.3237) (1.7562, 22.2686) knots 0 0 0 1 2 2 2
  spline S107 degree 2 poles (1.7562, 22.2686) (1.8161, 22.2184) (1.975, 22.1665) (2.0819, 22.1665) knots 0 0 0 1 2 2 2
  spline S108 degree 2 poles (2.0819, 22.1665) (2.1889, 22.1665) (2.3251, 22.2248) (2.3704, 22.28) knots 0 0 0 1 2 2 2
  spline S109 degree 2 poles (2.3704, 22.28) (2.4207, 22.3367) (2.4628, 22.5052) (2.4628, 22.6073) knots 0 0 0 1 2 2 2
  spline S110 degree 2 poles (2.4628, 22.6073) (2.4628, 22.7176) (2.4288, 22.9364) (2.4142, 23.0028) knots 0 0 0 1 2 2 2
  line L71 (2.4142, 23.0028) -> (3.445, 23.0028)
  line L72 (3.445, 23.0028) -> (3.445, 21.9056)
  line L73 (3.445, 21.9056) -> (3.21, 21.9056)
  line L74 (3.21, 21.9056) -> (3.21, 22.7451)
  line L75 (3.21, 22.7451) -> (2.6768, 22.7451)
  spline S111 degree 2 poles (2.6768, 22.7451) (2.6832, 22.6965) (2.6881, 22.6025) (2.6881, 22.5636) knots 0 0 0 1 2 2 2
  spline S112 degree 2 poles (2.6881, 22.5636) (2.6881, 22.4096) (2.6379, 22.1973) (2.5633, 22.1001) knots 0 0 0 1 2 2 2
  spline S113 degree 2 poles (2.5633, 22.1001) (2.4888, 22.0012) (2.2618, 21.8942) (2.0803, 21.8942) knots 0 0 0 1 2 2 2
  point P0 (0, 0)
  constraints: 4 other
extrude "Extrusion11" cut sketch "Sketch12" against normal blind 0.1
equation "\"d2\" = d5"
equation "\"d3\" = d5"
equation "\"d6\" = d5"
equation "\"d7\" = d5"
equation "\"d12\" = d5"
equation "\"d13\" = d5"
equation "\"d15\" = d5"
equation "\"d16\" = d5"
equation "\"d17\" = d5"
equation "\"d21\" = d11"
body "Solid1"
